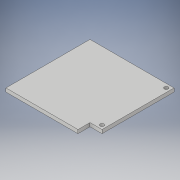
# Autodesk Inventor part: 000.109 - Правая боковая панель заднего сегмента
Saved by Autodesk Inventor 2019 (Build 230136000, 136)
## iProperties
Created: 2020-06-06
Part Number: 000.109 - Правая боковая панель заднего сегмента
Material: Типовые
Document SubType Name: Modeling
Designer: Петров Иван
Density: 1 g/cm^3
Appearance: По умолчанию
Author: Петров Иван
Autodesk Inventor part; units mm, degrees
ref_plane "YZ Plane" through (0, 0, 0) normal (1, 0, 0) x (0, 1, 0)
ref_plane "XZ Plane" through (0, 0, 0) normal (0, 1, 0) x (-1, 0, 0)
ref_plane "XY Plane" through (0, 0, 0) normal (0, 0, 1) x (1, 0, 0)
sketch "Эскиз1" plane through (0, 0, 0) normal (0, 1, 0) x (-1, 0, 0)
  line L0 (-35, 35) -> (35, 35)
  line L1 (35, 35) -> (35, -35)
  line L2 (35, -35) -> (-35, -35)
  line L3 (-35, -35) -> (-35, 35)
  line L4 (-35, 35) -> (35, -35) construction
  line L5 (35, 35) -> (-35, -35) construction
  line L6 (-35, 35) -> (-25, 35)
  line L7 (-25, 35) -> (-25, 25)
  line L8 (-25, 25) -> (-35, 25)
  line L9 (-35, 25) -> (-35, 35)
  circle A0 centre (-31.7678, 21.7678) radius 1.6
  line L10 (-35, -35) -> (-31.7678, -31.7678)
  circle A1 centre (-31.7678, -31.7678) radius 1.6
  point P0 (0, 0)
  point P1 (-35, 15)
  dimension "d0" = 70
  dimension "d1" = 70
  dimension "d3" = 10
  dimension "d5" = 3.2
  dimension "d7" = 4.571
  dimension "d8" = 3.2
  dimension "d11" = 4.5711
  dimension "d12" = 10
  constraints: 22 end point, 4 parallel, 2 centre point, 2 horizontal, 2 midpoint, 2 perpendicular, 2 point on line, 1 coincident
  measures "d0" distance of L1.end L2.end
  measures "d1" distance of L0.end L1.end
  measures "d3" distance of L6.end L7.end
  measures "d5" diameter of A0
  measures "d7" distance of L2.end L10.end
  measures "d8" diameter of A1
  measures "d11" distance of L8.end A0.centre
  measures "d12" distance of L7.end L8.end
extrude "Выдавливание1" add sketch "Эскиз1" along normal blind 3 contours L0 L1 L2 L3 L8 L7
